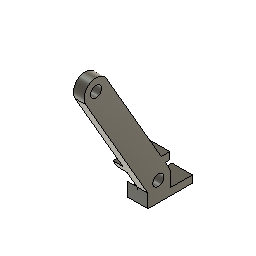
Speedo Sensor Bracket (Autodesk Fusion 360 design; units mm, degrees)
Autodesk Fusion 360 part; units mm, degrees
note: some values were not read from the file. Set by a fixed rule: which sketch regions a step uses.
sketch "Sensor Body" plane through (0, 0, 0) normal (0, 0, 1) x (1, 0, 0)
  line L0 (-11.43, -6.985) -> (0, -6.985)
  arc A0 (0, -6.985) -> (0, 6.985) centre (0, 0) ccw
  line L1 (0, 6.985) -> (-11.43, 6.985)
  arc A1 (-11.43, 6.985) -> (-11.43, -6.985) centre (-11.43, 0) ccw
  line L2 (-18.415, 0) -> (6.985, 0) construction
  circle A2 centre (0, 0) radius 5
  line L3 (-12.04, -3.05) -> (-10.82, -3.05)
  arc A3 (-10.82, -3.05) -> (-10.82, 3.05) centre (-10.82, 0) ccw
  line L4 (-10.82, 3.05) -> (-12.04, 3.05)
  arc A4 (-12.04, 3.05) -> (-12.04, -3.05) centre (-12.04, 0) ccw
  line L5 (-15.09, 0) -> (-7.77, 0) construction
  line L6 (-12.04, 0) -> (-10.82, 0)
  line L7 (5, 4.8775) -> (5, -4.8775)
  line L8 (-5, 4.8775) -> (-5, -4.8775)
  circle A5 centre (0, 0) radius 6.985
  point P0 (-11.43, 0)
  dimension "d1" = 13.97
  dimension "d2" = 10
  dimension "d3" = 6.1
  constraint tangent L0 A0
  constraint tangent A0 L1
  constraint parallel L0 L1
  constraint tangent L1 A1
  constraint tangent L0 A1
  constraint midpoint A1 L2.start
  constraint midpoint A0 L2.end
  constraint horizontal L2
  constraint concentric A0 A2
  constraint tangent L3 A3
  constraint tangent A3 L4
  constraint parallel L3 L4
  constraint tangent L4 A4
  constraint tangent L3 A4
  constraint midpoint A4 L5.start
  constraint midpoint A3 L5.end
  constraint horizontal L5
  constraint coincident A4.centre L6.start
  constraint coincident A3.centre L6.end
  constraint midpoint L6 P0
  constraint coincident P0 A1.centre
  constraint coincident A0.centre A2.centre
  constraint vertical L7
  constraint tangent A2 L7
  constraint perpendicular L0 L8
  constraint tangent A2 L8
  constraint coincident A0 L7.start
  constraint coincident A0 L7.end
  constraint concentric A2 A5
  constraint coincident A5 L8.start
  constraint coincident A5 L8.end
  measures "d1" diameter of A0
  measures "d2" diameter of A2
  measures "d3" diameter of A3
extrude "Extrude1" add sketch "Sensor Body" along normal blind 5.207 makes body 1
extrude "Extrude2" add sketch "Sensor Body" along normal blind 23.75 separate body contours A2 makes body 2
extrude "Extrude3" add sketch "Sensor Body" against normal blind 7.2 contours A0 A2 L7 L8 A5 | A0 A2 L7 L8 A5 | A2 bodies 1 2
ref_plane "WorkPlane2" through (-5.715, -6.985, 2.6035) normal (0, -1, 0) x (1, 0, 0)
sketch "Wire Placement" plane through (-5.715, -6.985, 2.6035) normal (0, -1, 0) x (1, 0, 0)
  line L0 (0.715, -9.8035) -> (10.715, -9.8035)
  line L1 (5.715, -2.6035) -> (5.715, -9.8035)
  point P0 (5.715, -2.6035)
  point P1 (5.715, -6.2035)
  constraint coincident P0 L1.start
  constraint midpoint L0 L1.end
  constraint midpoint L1 P1
ref_plane "WorkPlane1" through (-5.715, -6.985, 0) normal (0, 0.965926, 0.258819) x (1, 0, 0)
sketch "Wire Relief" plane through (-5.715, -6.985, 0) normal (0, 0.965926, 0.258819) x (1, 0, 0)
  circle A0 centre (5.715, 3.6157) radius 4.5
  point P0 (5.715, 3.6157)
  dimension "d12" = 9
  constraint coincident P0 A0.centre
  measures "d12" diameter of A0
extrude "Extrude4" add sketch "Wire Relief" along normal blind 4 bodies 1
extrude "Extrude5" cut sketch "Wire Relief" against normal blind 3 bodies 1
extrude "Extrude6" add sketch "Wire Relief" against normal blind 6.35 bodies 1
copy_body "Body->Comp1" bodies 1 removing the originals makes body 3 in component "Speed Sensor"
move_body "Move1" bodies 3 to x (0, 0, 1) y (0, 1, 0) z (-1, 0, 0) at (5.207, 0, 5.207) in component "Speed Sensor"
move_body "Move2" bodies 3 to x (1, 0, 0) y (0, 0, -1) z (0, 1, 0) at (0, 3.7047, 3.2243) in component "Speed Sensor"
sketch "Sketch1" plane through (0, 0, 0) normal (1, 0, 0) x (0, 1, 0) in component "Bracket"
  circle A0 centre (-3.1283, 3.2243) radius 3
  circle A1 centre (-38.1283, 63.846) radius 3
  line L0 (-3.1283, 3.2243) -> (-3.1283, 76.2225) construction
  arc A2 (-3.1283, 6.2743) -> (-3.1283, 0.1743) centre (-3.1283, 3.2243) ccw
  line L1 (-43.974, 60.471) -> (-8.974, -0.1507)
  arc A3 (-8.974, -0.1507) -> (2.7174, 6.5993) centre (-3.1283, 3.2243) ccw
  line L2 (2.7174, 6.5993) -> (-32.2826, 67.221)
  arc A4 (-32.2826, 67.221) -> (-43.974, 60.471) centre (-38.1283, 63.846) ccw
  line L3 (-38.1283, 63.846) -> (-3.1283, 3.2243) construction
  circle A5 centre (-3.1283, 3.2243) radius 3.1
  circle A6 centre (-38.1283, 63.846) radius 3.1
  line L4 (16.026, -7.7607) -> (-8.974, -7.7607)
  line L5 (8.9117, -3.7607) -> (-2.5183, -3.7607)
  line L6 (-8.974, -0.1507) -> (-8.974, -7.7607)
  line L7 (-3.1283, 3.2243) -> (3.6217, 3.2243) construction
  line L8 (3.6217, 3.2243) -> (3.6217, -3.7607)
  line L9 (16.026, -7.7607) -> (16.026, -3.7607)
  line L10 (16.026, -3.7607) -> (3.6217, -3.7607)
  line L11 (0.7781, 9.9581) -> (-14.8103, 9.9581)
  line L12 (0.7781, 9.9581) -> (3.2781, 9.9581)
  line L13 (3.2781, 9.9581) -> (3.2781, 13.9581)
  line L14 (3.2781, 13.9581) -> (-17.1197, 13.9581)
  line L15 (3.6217, -3.7607) -> (-6.1515, -3.7607)
  arc A7 (-8.974, -0.1507) -> (-6.1515, -3.7607) centre (-5.2541, -0.1507) ccw
  point P0 (3.6217, 3.2243)
  dimension "d19" = 6
  dimension "d20" = 6
  dimension "d21" = 70
  dimension "d23" = 13.5
  dimension "d24" = 6.2
  dimension "d25" = 6.2
  dimension "d26" = 4
  dimension "d27" = 25
  dimension "d28" = 4
  dimension "d29" = 2.5
  dimension "d30" = 4
  dimension "d36" = 30
  constraint coincident A0.centre L0.start
  constraint vertical L0
  constraint concentric A0 A2
  constraint tangent L1 A3
  constraint tangent A3 L2
  constraint parallel L1 L2
  constraint tangent L2 A4
  constraint tangent L1 A4
  constraint coincident A1.centre A4.centre
  constraint concentric A0 A5
  constraint concentric A1 A6
  constraint horizontal L4
  constraint coincident L4 L6.end
  constraint perpendicular L4 L6
  constraint coincident L4.end L6.end
  constraint coincident A3 P0
  constraint perpendicular L0 L7
  constraint coincident P0 L7.end
  constraint tangent A3 L8
  constraint perpendicular L4 L9
  constraint coincident L5 L8.end
  constraint coincident L2 L11.start
  constraint coincident L1 L11.end
  constraint perpendicular L0 L11
  constraint parallel L11 L12
  constraint perpendicular L12 L13
  constraint coincident L1 L14.end
  constraint perpendicular L0 L14
  constraint perpendicular L8 L15
  constraint tangent L6 A7
  measures "d19" diameter of A0
  measures "d20" diameter of A1
  measures "d21" distance of A0.centre A1.centre
  measures "d23" diameter of A3
  measures "d24" diameter of A5
  measures "d25" diameter of A6
  measures "d26" distance of L4 L5
  measures "d27" distance of L4.start L4.end
  measures "d28" distance of L4.start L9.end
  measures "d29" distance of L11.start L12.end
  measures "d30" distance of L12.end L13.end
  measures "d36" angle of L0 L2
extrude "Extrude1'" add sketch "Sketch1" along normal blind 6 separate body contours L1 L2 A4 L14 | L1 L2 L11 L14 | L1 A3 L2 L11 | L2 L12 L13 L14 | L4 L5 L6 L9 L10 L15 A7 | A3 L5 L8 L15 A7 makes body 4 in component "Bracket"
extrude "Extrude2'" add sketch "Sketch1" against normal blind 5.5 contours L1 L2 L11 L14 | L2 L12 L13 L14 | L4 L5 L6 L9 L10 L15 A7 bodies 4 in component "Bracket"
component "Speed Sensor" placed x (1, 0, 0) y (0, 1, 0) z (0, 0, 1) at (0, 0, 0)
component "Bracket" placed x (1, 0, 0) y (0, 1, 0) z (0, 0, 1) at (0, 0, 0)
equation "d24 = MountingHole"
equation "d25 = MountingHole"
equation "d31 = BracketThickness"
equation "MountingHole = 6.2 mm"
equation "d36 = BracketAngle"
equation "BracketAngle = 30 deg"
equation "BracketThickness = 6 mm"
named bodies: "Speed Sensor"
